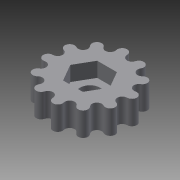
# Autodesk Inventor part: knurled nut
Saved by Autodesk Inventor 2015 SP2 (Build 190223200, 223)
## iProperties
Created: 2015-05-21
Part Number: knurled nut
Material: Generic
Document SubType Name: Modeling
Designer: caleb
Density: 1 g/cm^3
Appearance: Default
Author: caleb
Autodesk Inventor part; units mm, degrees
ref_plane "YZ Plane" through (0, 0, 0) normal (1, 0, 0) x (0, 1, 0)
ref_plane "XZ Plane" through (0, 0, 0) normal (0, 1, 0) x (-1, 0, 0)
ref_plane "XY Plane" through (0, 0, 0) normal (0, 0, 1) x (1, 0, 0)
sketch "Sketch1" plane through (0, 0, 0) normal (0, 0, 1) x (1, 0, 0)
  line L0 (3.3198, 5.75) -> (6.6395, 0)
  line L1 (6.6395, 0) -> (3.3198, -5.75)
  line L2 (3.3198, -5.75) -> (-3.3198, -5.75)
  line L3 (-3.3198, -5.75) -> (-6.6395, 0)
  line L4 (-6.6395, 0) -> (-3.3198, 5.75)
  line L5 (-3.3198, 5.75) -> (3.3198, 5.75)
  circle A0 centre (0, 0) radius 12.5
  dimension "d0" = 11.5
  dimension "d1" = 25
  constraints: 12 end point, 2 coincident, 1 centre point, 1 horizontal, 13 other
  measures "d0" distance between parallel lines of L2 L5
  measures "d1" diameter of A0
extrude "Extrusion1" add sketch "Sketch1" against normal blind 5
sketch "Sketch2" plane through (0, 0, -5) normal (0, 0, -1) x (-1, 0, 0)
  circle A0 centre (0, 0) radius 12.5 projected
extrude "Extrusion2" add sketch "Sketch2" along normal blind 3
sketch "Sketch3" plane through (0, 0, -8) normal (0, 0, -1) x (-1, 0, 0)
  circle A0 centre (0, 0) radius 12.5 construction
hole "Hole1" at (0, 0, -8) direction (0, 0, 1) diameter 6.756 end through all clearance for "Flat Head Machine Screw (82)" size "1/4" standard "Ansi Unified Screw Threads"
sketch "Sketch4" plane through (0, 0, 0) normal (0, 0, 1) x (1, 0, 0)
  circle A0 centre (0, 0) radius 12.5 projected
  arc A1 (0, 12.5) -> (3.2352, 12.0741) centre (1.6457, 12.5) ccw
  arc A2 (6.25, 10.8253) -> (3.2352, 12.0741) centre (4.8248, 11.6481) ccw
  line L0 (0, 12.5) -> (0, 0) construction
  line L1 (-6.25, 10.8253) -> (0, 0) construction
  line L2 (-10.8253, 6.25) -> (0, 0) construction
  line L3 (-12.5, 0) -> (0, 0) construction
  line L4 (-10.8253, -6.25) -> (0, 0) construction
  line L5 (-6.25, -10.8253) -> (0, 0) construction
  line L6 (0, -12.5) -> (0, 0) construction
  line L7 (6.25, -10.8253) -> (0, 0) construction
  line L8 (10.8253, -6.25) -> (0, 0) construction
  line L9 (12.5, 0) -> (0, 0) construction
  line L10 (10.8253, 6.25) -> (0, 0) construction
  line L11 (6.25, 10.8253) -> (0, 0) construction
  dimension "d15" = 360
  constraints: 24 end point, 7 point on circle, 2 centre point, 2 tangent, 1 coincident, 1 equal radius, 1 vertical, 1 vertical alignment, 37 other
extrude "Extrusion3" cut sketch "Sketch4" against normal through all contours A0 A1 picked at (1.5636, 11.877)
extrude "Extrusion4" add sketch "Sketch4" against normal up to surface (8 mm away) contours A0 A2
pattern_circular "Circular Pattern1" count 12 over 360 about axis through (0, 0, -10) along (0, 0, 1) of "Extrusion3", "Extrusion4"
body "Solid1"
